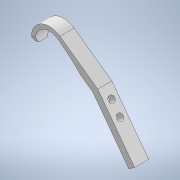
# Autodesk Inventor part: foot_1
Saved by Autodesk Inventor 2020 (Build 240168000, 168)
## iProperties
Created: 2020-12-13
Part Number: foot_1
Material: Generic
Document SubType Name: Modeling
Designer: Shuang Peng
Density: 1 g/cm^3
Appearance: Default
Author: Shuang Peng
Autodesk Inventor part; units mm, degrees
ref_plane "YZ Plane" through (0, 0, 0) normal (1, 0, 0) x (0, 1, 0)
ref_plane "XZ Plane" through (0, 0, 0) normal (0, 1, 0) x (-1, 0, 0)
ref_plane "XY Plane" through (0, 0, 0) normal (0, 0, 1) x (1, 0, 0)
sketch "Sketch1" plane through (0, 0, 0) normal (0, 0, 1) x (1, 0, 0)
  circle A0 centre (21.6472, -15.01) radius 3.075 projected
  circle A1 centre (-9.3299, 6.9995) radius 3.075 projected
  line L0 (-25.0169, 15.9984) -> (-22.9897, 18.8516) projected
  line L1 (-25.0169, 15.9984) -> (-15.1619, 8.9964) projected
  arc A2 (-14.323, 7.2613) -> (-15.1619, 8.9964) centre (-16.3203, 7.366) ccw projected
  arc A3 (-14.323, 7.2613) -> (-7.4396, 2.3706) centre (-9.3299, 6.9995) ccw projected
  arc A4 (-5.5251, 2.1494) -> (-7.4396, 2.3706) centre (-6.6835, 0.519) ccw projected
  line L2 (-5.5251, 2.1494) -> (15.8152, -13.0131) projected
  arc A5 (16.6541, -14.7482) -> (15.8152, -13.0131) centre (14.6569, -14.6434) ccw projected
  arc A6 (16.6541, -14.7482) -> (19.7569, -10.3811) centre (21.6472, -15.01) ccw projected
  arc A7 (17.8424, -10.1599) -> (19.7569, -10.3811) centre (19.0008, -8.5295) ccw projected
  line L3 (17.8424, -10.1599) -> (-3.4979, 5.0025) projected
  arc A8 (-4.3368, 6.7377) -> (-3.4979, 5.0025) centre (-2.3395, 6.6329) ccw projected
  arc A9 (-4.3368, 6.7377) -> (-11.2202, 11.6284) centre (-9.3299, 6.9995) ccw projected
  arc A10 (-13.1347, 11.8496) -> (-11.2202, 11.6284) centre (-11.9763, 13.4799) ccw projected
  line L4 (-13.1347, 11.8496) -> (-22.9897, 18.8516) projected
  line L5 (-26.6472, 17.1568) -> (-25.0169, 15.9984) projected
  line L6 (-25.0169, 15.9984) -> (-22.9897, 18.8516) projected
  line L7 (-22.9897, 18.8516) -> (-24.6201, 20.01) projected
  line L8 (-24.6201, 20.01) -> (-26.6472, 17.1568) projected
  line L9 (-17.6802, 10.7857) -> (-15.653, 13.6388)
  line L10 (-15.653, 13.6388) -> (-13.2074, 11.9012)
  line L11 (-13.2074, 11.9012) -> (-11.1802, 14.7544)
  line L12 (-11.1802, 14.7544) -> (-39.7118, 35.0263)
  line L13 (-39.7118, 35.0263) -> (-50.1374, 20.3529)
  arc A11 (-39.7118, 35.0263) -> (-50.1374, 20.3529) centre (-44.9246, 27.6896) ccw
  line L14 (-50.1374, 20.3529) -> (-48.979, 21.9833)
  line L15 (-48.979, 21.9833) -> (-40.8702, 33.3959)
  arc A12 (-40.8702, 33.3959) -> (-48.979, 21.9833) centre (-44.9246, 27.6896) ccw
  line L16 (-15.653, 13.6388) -> (-41.739, 32.1731)
  point P0 (0, 0)
  dimension "d0" = 3
  dimension "d1" = 3.5
  dimension "d2" = 35
  dimension "d5" = 18
  dimension "d6" = 2
  dimension "d7" = 14
  constraints: 16 end point, 4 point on circle, 4 point on line, 3 perpendicular, 2 centre point, 2 midpoint, 1 parallel, 3 other
  measures "d0" distance of L9.end L10.end
  measures "d1" distance of L10.end L11.end
  measures "d2" distance of L11.end L12.end
  measures "d5" distance of L12.end L13.end
  measures "d6" distance of L13.end L14.end
  measures "d7" distance of L14.end L15.end
ref_plane "Work Plane1" through (-42.7768, -43.6207, -7) normal (0, 0, -1) x (0, 1, 0)
extrude "Extrusion1" add sketch "Sketch1" against normal up to surface (7 mm away) contours L7 L16 L13 L12 L11 L4 | A12 L13 A11
sketch "Sketch3" plane through (-11.1802, 14.7544, -7) normal (0, 0, -1) x (-0.8151879, 0.5791965, 0)
  arc A0 (35, -18) -> (35, 0) centre (35, -9) ccw projected
  line L0 (0, 0) -> (35, 0) projected
  line L1 (0, -3.5) -> (0, 0) projected
  line L2 (35, -3.5) -> (0, -3.5) projected
  line L3 (35, -2) -> (35, -3.5) projected
  arc A1 (35, -16) -> (35, -2) centre (35, -9) ccw projected
  line L4 (35, -3.5) -> (0, -3.5) projected
  line L5 (35, -3.5) -> (20, -3.5)
  line L6 (35, -2) -> (35, -3.5) projected
  arc A2 (35, -2) -> (20, -3.5) centre (35, -77.75) ccw
  line L7 (35, -18) -> (35, -16) projected
  point P0 (-17.6597, -5.552)
  point P1 (20, -3.5)
  dimension "d17" = 15
  constraints: 2 end point, 2 point on circle, 1 centre point, 1 line through centre, 1 point on line
  measures "d17" distance of L2.start L5.end
extrude "Extrusion3" cut sketch "Sketch3" against normal blind 10 contours L3 L2 A2
thicken "Thicken1" operation add thickness 12 both sides no extend neighbours yes toward (-0.8151879, 0.5791965, 0) faces at (-12.5317, 12.8523, -2.3333)
sketch "Sketch4" plane through (-44.9246, 27.6896, -7) normal (0, 0, -1) x (-0.8151879, 0.5791965, 0)
  arc A0 (0, 7) -> (-15, 5.5) centre (0, -68.75) ccw projected
  arc A1 (0, -7) -> (0, 7) centre (0, 0) ccw projected
  line L0 (0, -9) -> (0, -7) projected
  arc A2 (0, -9) -> (0, 9) centre (0, 0) ccw projected
  line L1 (-23, 9) -> (0, 9) projected
  line L2 (-23, 5.5) -> (-23, 9) projected
  line L3 (-15, 5.5) -> (-23, 5.5) projected
  line L4 (-22.4457, 5.5) -> (-50.9773, -3.7705)
  line L5 (-23, 9) -> (0, 9) projected
  line L6 (-23, 9) -> (-52.0589, -0.4418)
  line L7 (-50.9773, -3.7705) -> (-52.0589, -0.4418)
  point P0 (-52.6597, 3.448)
  point P1 (-18.4769, 9)
  dimension "d22" = 30
  dimension "d23" = 108
  dimension "d24" = 3.5
  constraints: 6 end point, 1 parallel, 1 perpendicular, 1 point on line
  measures "d22" distance of L4.start L4.end
  measures "d23" angle of L2 L4
  measures "d24" distance between parallel lines of L4 L6
extrude "Extrusion4" add sketch "Sketch4" against normal up to surface (7 mm away) contours L4 L7 L6 L2 L3
sketch "Sketch5" plane through (-44.9246, 27.6896, -7) normal (0, 0, -1) x (-0.8151879, 0.5791965, 0)
  arc A0 (0, 7) -> (-15, 5.5) centre (0, -68.75) ccw projected
  arc A1 (0, -7) -> (0, 7) centre (0, 0) ccw projected
  line L0 (0, -9) -> (0, -7) projected
  arc A2 (0, -9) -> (0, 9) centre (0, 0) ccw projected
  line L1 (-23, 9) -> (0, 9) projected
  line L2 (-23, 9) -> (-52.0589, -0.4418) projected
  line L3 (-52.0589, -0.4418) -> (-50.9773, -3.7705) projected
  line L4 (-50.9773, -3.7705) -> (-22.4457, 5.5) projected
  line L5 (-15, 5.5) -> (-22.4457, 5.5) projected
  line L6 (0, 0) -> (0, -9)
  line L7 (0, 0) -> (5.7851, -6.8944)
  arc A3 (0, -9) -> (0, 9) centre (0, 0) ccw projected
  point P0 (-52.6597, 3.448)
  point P1 (5.7851, -6.8944)
  point P2 (4.4995, -5.3623)
  dimension "d27" = 40
  constraints: 4 end point, 1 point on circle, 1 vertical
  measures "d27" angle of L6 L7
extrude "Extrusion5" cut sketch "Sketch5" against normal blind 10 contours L7 A2 L0 A1
chamfer "Chamfer2" distance 1.5 angle 60 2 edges at (-52.6661, 25.6722, -7) (-52.6661, 25.6722, 0) measured on face at (-52.6661, 25.6722, -6.5) measured on face at (-52.6661, 25.6722, -0.5)
sketch "Sketch6" plane through (-23.4416, 19.1727, -7) normal (-0.8027556, -0.5963082, 0) x (0, 0, 1)
  line L0 (7, -30) -> (7, 0) projected
  line L1 (0, 0) -> (7, 0) projected
  line L2 (0, -30) -> (0, 0) projected
  line L3 (0, -30) -> (7, -30) projected
  line L4 (0, 0) -> (7, 0) projected
  line L5 (3.5, 0) -> (3.5, -6)
  line L6 (3.5, -6) -> (3.5, -13)
  circle A0 centre (3.5, -6) radius 1.6
  circle A1 centre (3.5, -13) radius 1.6
  point P0 (7, -29.3694)
  dimension "d33" = 6
  dimension "d34" = 7
  dimension "d35" = 3.2
  dimension "d36" = 3.2
  constraints: 4 end point, 2 centre point, 2 coincident, 2 parallel, 1 midpoint
  measures "d33" distance of L5.start L5.end
  measures "d34" distance of L5.end L6.end
  measures "d35" diameter of A0
  measures "d36" diameter of A1
extrude "Extrusion6" cut sketch "Sketch6" against normal blind 10 contours A0 L6 L5 | L5 L6 A0 | A1
thicken "Thicken2" operation add thickness 13 both sides no extend neighbours yes toward (-0.5963082, 0.8027556, 0) faces at (-3.6792, -3.5186, -4.6667)
chamfer "Chamfer3" distance 2 angle 45 2 edges at (-11.8995, 6.5694, -7) (-11.8995, 6.5694, 0)
thicken "Thicken3" operation add thickness 0.5 both sides no extend neighbours yes toward (-0.8027556, -0.5963082, 0) faces at (-19.9754, 20.3759, -3.5643)
fillet "Fillet1" radius 8 2 edges at (-22.2815, 22.6419, -3.5) (-23.4416, 19.1727, -3.5)
fillet "Fillet2" radius 20 1 edges at (-29.5112, 23.4852, -3.5)
body "Solid1"
